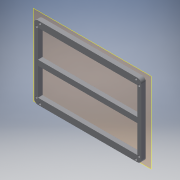
# Autodesk Inventor part: Omniscope_Lid
Saved by Autodesk Inventor 2019.4 (Build 234330000, 330)
## iProperties
Created: 2021-10-01
Part Number: Omniscope_Lid
Material: Generic
Document SubType Name: Modeling
Designer: diederichbenedict
Density: 1 g/cm^3
Appearance: Default
Author: diederichbenedict
Autodesk Inventor part; units mm, degrees
ref_plane "YZ Plane" through (0, 0, 0) normal (1, 0, 0) x (0, 1, 0)
ref_plane "XZ Plane" through (0, 0, 0) normal (0, 1, 0) x (-1, 0, 0)
ref_plane "Work Plane1" through (0, 0, 0) normal (0, 0, 1) x (1, 0, 0)
sketch "Sketch1" plane through (0, 0, 0) normal (0, 0, 1) x (1, 0, 0)
  circle A0 centre (-56, 33.5) radius 1.35 projected
  circle A1 centre (-52.5, -38) radius 1.35 projected
  circle A2 centre (56, -33.5) radius 1.35 projected
  circle A3 centre (52.5, 38) radius 1.35 projected
  circle A4 centre (56, 33.5) radius 1.35 projected
  circle A5 centre (52.5, -38) radius 1.35 projected
  circle A6 centre (-56, -33.5) radius 1.35 projected
  circle A7 centre (-52.5, 38) radius 1.35 projected
  line L0 (-54.4, 35.9) -> (54.4, 35.9) projected
  line L1 (54.4, 35.9) -> (54.4, -35.9) projected
  line L2 (54.4, -35.9) -> (-54.4, -35.9) projected
  line L3 (-54.4, -35.9) -> (-54.4, 35.9) projected
  arc A8 (-58.5, -36) -> (-54.5, -40) centre (-54.5, -36) ccw projected
  line L4 (-54.5, -40) -> (54.5, -40) projected
  arc A9 (54.5, -40) -> (58.5, -36) centre (54.5, -36) ccw projected
  line L5 (58.5, -36) -> (58.5, 36) projected
  arc A10 (58.5, 36) -> (54.5, 40) centre (54.5, 36) ccw projected
  line L6 (54.5, 40) -> (-54.5, 40) projected
  arc A11 (-54.5, 40) -> (-58.5, 36) centre (-54.5, 36) ccw projected
  line L7 (-58.5, 36) -> (-58.5, -36) projected
  line L8 (36.5917, -33) -> (54.3917, -33) construction
  line L9 (54.3917, -3.2) -> (54.3917, -33) construction
  line L10 (54.3917, -3.2) -> (36.5917, -3.2) construction
  line L11 (36.5917, -33) -> (36.5917, -3.2) construction
  circle A12 centre (45.4917, -9.15) radius 3.375 construction
  circle A13 centre (45.4917, -27.05) radius 3.375 construction
  circle A14 centre (50.9917, -18.1) radius 3 construction
  circle A15 centre (39.9917, -18.1) radius 3 construction
  circle A16 centre (45.4917, -18.1) radius 1.4 construction
  line L12 (36.5917, 3) -> (54.3917, 3) construction
  line L13 (54.3917, 32.8) -> (54.3917, 3) construction
  line L14 (54.3917, 32.8) -> (36.5917, 32.8) construction
  line L15 (36.5917, 3) -> (36.5917, 32.8) construction
  circle A17 centre (45.4917, 26.85) radius 3.375 construction
  circle A18 centre (45.4917, 8.95) radius 3.375 construction
  circle A19 centre (50.9917, 17.9) radius 3 construction
  circle A20 centre (39.9917, 17.9) radius 3 construction
  circle A21 centre (45.4917, 17.9) radius 1.4 construction
  line L16 (54.4, -35.9) -> (-55.0436, -35.9)
  line L17 (-55.0436, -35.9) -> (-55.0436, -33.2)
  line L18 (-55.0436, -33.2) -> (54.4, -33.2)
  line L19 (54.4, -33.2) -> (54.4, -35.9)
  line L20 (54.4, 35.9) -> (-54.4, 35.9)
  line L21 (-54.4, 35.9) -> (-54.4, 33)
  line L22 (-54.4, 33) -> (54.4, 33)
  line L23 (54.4, 33) -> (54.4, 35.9)
  line L24 (54.4, -3) -> (-54.4, -3)
  line L25 (-54.4, -3) -> (-54.4, 2.8)
  line L26 (-54.4, 2.8) -> (54.4, 2.8)
  line L27 (54.4, 2.8) -> (54.4, -3)
  point P0 (0, 0)
  dimension "d0" = 0.2
  dimension "d1" = 0.2
  dimension "d2" = 0.2
  dimension "d3" = 0.2
  constraints: 24 end point, 6 parallel, 3 horizontal, 3 perpendicular, 3 point on line
  measures "d0" distance between parallel lines of L18 L8
  measures "d1" distance between parallel lines of L14 L22
  measures "d2" distance between parallel lines of L12 L26
  measures "d3" distance between parallel lines of L10 L24
ref_plane "Work Plane2" through (18.5917, -33, 5) normal (0, 0, 1) x (1, 0, 0)
extrude "Extrusion1" add sketch "Sketch1" along normal up to surface (5 mm away) contours A6 L17 L18 | A6 L18 L3 L16 L17 | L18 L1 L2 L3 | L3 L26 L1 L24 | L3 L0 L1 L22 | L7 A11 L6 A10 L5 A9 L4 A8 picked at (-54.9879, -33.9671)
body "Solid1"
